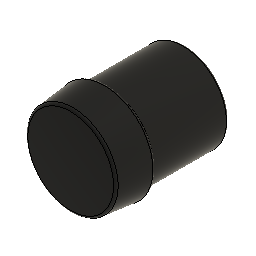
20021-016_payload-rod-cap (Autodesk Fusion 360 design; units mm, degrees)
Autodesk Fusion 360 part; units mm, degrees
sketch "Sketch1" plane through (0, 0, 0) normal (1, 0, 0) x (0, 1, 0)
  line L0 (0, 0) -> (0, 4.6)
  line L1 (0, 4.6) -> (3.7, 5)
  line L2 (3.7, 5) -> (3.7, 4.455)
  line L3 (3.7, 4.455) -> (11.7, 4.455)
  line L4 (11.7, 4.455) -> (11.7, 0)
  line L5 (11.7, 0) -> (0, 0)
  dimension "d1" = 4.455
  dimension "d2" = 3.7
  dimension "d3" = 5
  dimension "d4" = 4.6
  dimension "d5" = 8
  constraint coincident L0.start L5.end
  constraint vertical L0
  constraint parallel L0 L2
  constraint perpendicular L0 L3
  constraint perpendicular L3 L4
  constraint perpendicular L0 L5
  measures "d1" distance of L3.end L4.end
  measures "d2" distance of L0 L2
  measures "d3" distance of L1.end L5
  measures "d4" distance of L0.end L5
  measures "d5" distance of L2.end L3.end
revolve "Revolve1" add sketch "Sketch1" angle 360 about axis through (0, 11.7, 0) along (0, -1, 0)
fillet "Fillet1" radius 0.25 5 faces at (2.1309, 2.8778, 4.4248) (0.4697, 3.7, 4.7831) (0.2221, 6.3667, 4.4495) (0.3414, 11.7, 0.134) (0.0152, 0, -1.4325)
equation "d1 = ( 8.91 / 2 ) * 1 mm"
equation "d4 = ( 9.2 / 2 ) * 1 mm"
